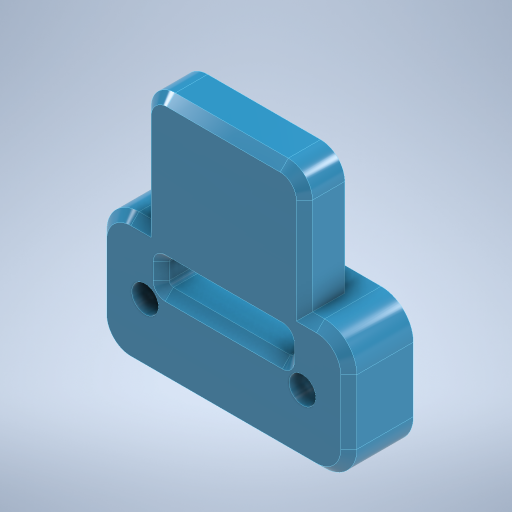
# Autodesk Inventor part: Base_VL53L0X
Saved by Autodesk Inventor 2024 (Build 280153000, 153)
## iProperties
Created: 2023-11-04
Part Number: Base_VL53L0X
Material: Generic
Document SubType Name: Modeling
Designer: fredy
Density: 1 g/cm^3
Appearance: Sky Blue Dark
Author: fredy
Autodesk Inventor part; units mm, degrees
ref_plane "YZ Plane" through (0, 0, 0) normal (1, 0, 0) x (0, 1, 0)
ref_plane "XZ Plane" through (0, 0, 0) normal (0, 1, 0) x (-1, 0, 0)
ref_plane "XY Plane" through (0, 0, 0) normal (0, 0, 1) x (1, 0, 0)
sketch "Sketch3" plane through (0, 0, 0) normal (0, 0, 1) x (1, 0, 0)
  line L0 (0, -11.2) -> (0, 11.2) projected
  line L1 (15.5, -8) -> (-15.5, -8)
  line L2 (-15.5, -8) -> (-15.5, 8)
  line L3 (-15.5, 8) -> (15.5, 8)
  line L4 (15.5, 8) -> (15.5, -8)
  line L5 (15.5, -8) -> (-15.5, 8) construction
  line L6 (-15.5, -8) -> (15.5, 8) construction
  point P0 (0, 0)
  dimension "d45" = 16
  dimension "d46" = 31
  constraints: 12 end point, 2 midpoint, 2 parallel, 1 horizontal, 1 perpendicular
  measures "d45" distance of L3.end L1.start
  measures "d46" distance of L2.end L3.end
extrude "Extrusion2" add sketch "Sketch3" along normal blind 4
sketch "Sketch5" plane through (0, 0, 4) normal (0, 0, 1) x (1, 0, 0)
  line L0 (-7.75, 2) -> (7.75, 2)
  line L1 (7.75, 2) -> (7.75, 5)
  line L2 (7.75, 5) -> (-7.75, 5)
  line L3 (-7.75, 5) -> (-7.75, 2)
  line L4 (-7.75, 2) -> (7.75, 5) construction
  line L5 (7.75, 2) -> (-7.75, 5) construction
  point P0 (0, 0)
  point P1 (0, 3.5)
  dimension "d33" = 3
  dimension "d36" = 2
  dimension "d37" = 15.5
  constraints: 12 end point, 2 midpoint, 2 parallel, 1 horizontal, 1 perpendicular, 1 vertical alignment
  measures "d33" distance of L2.end L0.start
  measures "d36" distance from line of point (0, 0) L0
  measures "d37" distance of L1.end L2.end
extrude "Extrusion3" cut sketch "Sketch5" against normal up to surface (4 mm away)
fillet "Fillet4" radius 0.5 4 edges at (7.75, 2, 2) (-7.75, 2, 2) (-7.75, 5, 2) (7.75, 5, 2)
fillet "Fillet5" radius 4 4 edges at (-15.5, 8, 2) (15.5, 8, 2) (15.5, -8, 2) (-15.5, -8, 2)
sketch "Sketch9" plane through (0, 0, 0) normal (0, 0, -1) x (-1, 0, 0)
  line L0 (-15.5, -4) -> (-15.5, 4) projected
  arc A0 (-11.5, 8) -> (-15.5, 4) centre (-11.5, 4) ccw projected
  line L1 (-11.5, 8) -> (11.5, 8) projected
  arc A1 (15.5, 4) -> (11.5, 8) centre (11.5, 4) ccw projected
  line L2 (15.5, 4) -> (15.5, -4) projected
  arc A2 (11.5, -8) -> (15.5, -4) centre (11.5, -4) ccw projected
  line L3 (11.5, -8) -> (-11.5, -8) projected
  arc A3 (-15.5, -4) -> (-11.5, -8) centre (-11.5, -4) ccw projected
  line L4 (-11.5, -6) -> (11.5, -6)
  line L5 (13.5, -4) -> (13.5, 4)
  line L6 (11.5, 6) -> (-11.5, 6)
  line L7 (-13.5, 4) -> (-13.5, -4)
  line L8 (-13.5, -6) -> (13.5, 6) construction
  line L9 (13.5, -6) -> (-13.5, 6) construction
  arc A4 (-11.5, 6) -> (-13.5, 4) centre (-11.5, 4) ccw
  arc A5 (-13.5, -4) -> (-11.5, -6) centre (-11.5, -4) ccw
  arc A6 (11.5, -6) -> (13.5, -4) centre (11.5, -4) ccw
  arc A7 (13.5, 4) -> (11.5, 6) centre (11.5, 4) ccw
  point P0 (0, 0)
  dimension "d59" = 2
  constraints: 12 end point, 8 point on circle, 8 point on line, 8 tangent, 4 centre point, 3 equal radius, 2 midpoint, 2 parallel, 1 coincident, 1 horizontal, 1 perpendicular
  measures "d59" radius of A4
extrude "Extrusion5" add sketch "Sketch9" along normal blind 4
sketch "Sketch11" plane through (0, 0, 0) normal (0, 0, -1) x (-1, 0, 0)
  circle A0 centre (-9.75, 0) radius 2.5
  line L0 (0, -11.2) -> (0, 11.2) projected
  circle A1 centre (9.75, 0) radius 2.5
  point P0 (0, 0)
  dimension "d63" = 19.5
  dimension "d64" = 5
  constraints: 2 centre point, 1 horizontal alignment, 1 symmetric about line, 1 other
  measures "d63" distance of A1.centre A0.centre
  measures "d64" diameter of A0
extrude "Extrusion7" add sketch "Sketch11" along normal blind 1.5
sketch "Sketch12" plane through (0, 0, 4) normal (0, 0, 1) x (1, 0, 0)
  line L0 (0, -11.2) -> (0, 11.2) projected
  point P0 (0, 0)
  point P1 (-9.75, 0)
  point P2 (9.75, 0)
  dimension "d67" = 19.5
  constraints: 1 horizontal alignment, 1 symmetric about line
  measures "d67" distance of point (9.75, 0) point (-9.75, 0)
hole "Hole4" at (-9.75, 0, 4) at (9.75, 0, 4) direction (0, 0, -1) diameter 3.3 end through all
fillet "Fillet6" radius 1 2 edges at (12.25, 0, 0) (-7.25, 0, 0)
sketch "Sketch13" plane through (-11.5, 8, 4) normal (0, 1, 0) x (1, 0, 0)
  line L0 (1.5, 0) -> (21.5, 0)
  line L1 (21.5, 0) -> (21.5, 5)
  line L2 (21.5, 5) -> (1.5, 5)
  line L3 (1.5, 5) -> (1.5, 0)
  line L4 (1.5, 0) -> (21.5, 5) construction
  line L5 (21.5, 0) -> (1.5, 5) construction
  line L6 (23, 0) -> (0, 0) projected
  point P0 (11.5, 4)
  point P1 (11.5, 2.5)
  point P2 (11.5, 0)
  dimension "d76" = 20
  dimension "d77" = 5
  constraints: 12 end point, 4 midpoint, 2 parallel, 1 horizontal, 1 perpendicular
  measures "d76" distance of L1.end L2.end
  measures "d77" distance of L2.end L0.start
extrude "Extrusion8" add sketch "Sketch13" along normal blind 15
fillet "Fillet7" radius 3 2 edges at (-10, 23, 1.5) (10, 23, 1.5)
chamfer "Chamfer1" distance 1 angle 45 22 edges at (-10, 14, 4) (-9.1213, 22.1213, 4) (0, 23, 4) (9.1213, 22.1213, 4) (10, 14, 4) (0, -8, 4) (14.3284, -6.8284, 4) (15.5, 0, 4) (14.3284, 6.8284, 4) (10.75, 8, 4) (-14.3284, -6.8284, 4) (-15.5, 0, 4) (-14.3284, 6.8284, 4) (-10.75, 8, 4) (0, 5, 4) (7.6036, 4.8536, 4) (7.75, 3.5, 4) (7.6036, 2.1464, 4) (0, 2, 4) (-7.6036, 2.1464, 4) (-7.75, 3.5, 4) (-7.6036, 4.8536, 4)
body "Solid2"
